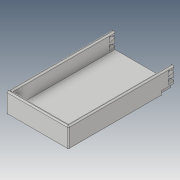
# Autodesk Inventor part: Case_metà1
Saved by Autodesk Inventor 2019 (Build 230136000, 136)
## iProperties
Created: 2019-05-06
Part Number: Case_metà1
Material: Generic
Document SubType Name: Modeling
Designer: giacomo
Density: 1 g/cm^3
Appearance: Default
Author: giacomo
Autodesk Inventor part; units mm, degrees
ref_plane "YZ Plane" through (0, 0, 0) normal (1, 0, 0) x (0, 1, 0)
ref_plane "XZ Plane" through (0, 0, 0) normal (0, 1, 0) x (-1, 0, 0)
ref_plane "XY Plane" through (0, 0, 0) normal (0, 0, 1) x (1, 0, 0)
sketch "Sketch1" plane through (0, 0, 0) normal (0, 1, 0) x (-1, 0, 0)
  line L0 (-50, 75) -> (50, 75)
  line L1 (50, 75) -> (50, -75)
  line L2 (50, -75) -> (-50, -75)
  line L3 (-50, -75) -> (-50, 75)
  line L4 (-50, 75) -> (50, -75) construction
  line L5 (50, 75) -> (-50, -75) construction
  point P0 (0, 0)
  dimension "d0" = 100
  dimension "d1" = 150
  constraints: 12 end point, 2 midpoint, 2 parallel, 1 horizontal, 1 perpendicular
  measures "d0" distance of L1.end L2.end
  measures "d1" distance of L0.end L1.end
extrude "Extrusion1" add sketch "Sketch1" along normal blind 8
sketch "Sketch3" plane through (0, 8, 0) normal (0, 1, 0) x (1, 0, 0)
  line L0 (-50, -75) -> (50, -75) projected
  line L1 (50, -75) -> (50, 75) projected
  line L2 (50, 75) -> (-50, 75) projected
  line L3 (-50, 75) -> (-50, -75) projected
  line L4 (45, 75) -> (45, -70)
  line L5 (-50, -75) -> (50, -75) projected
  line L6 (50, -75) -> (50, 75) projected
  line L7 (0, 0) -> (0, -83) construction
  line L8 (-45, 75) -> (-45, -70)
  line L9 (45, -70) -> (-45, -70)
  dimension "d4" = 5
  dimension "d5" = 5
  constraints: 8 end point, 3 parallel, 2 point on line, 1 perpendicular, 1 vertical, 1 other
  measures "d4" distance between parallel lines of L1 L4
  measures "d5" distance between parallel lines of L9 L0
extrude "Extrusion2" add sketch "Sketch3" along normal blind 25 contours L3 L2 L8 L9 L4 L1 L0
sketch "Sketch4" plane through (50, 0, -75) normal (0, 0, -1) x (-1, 0, 0)
  line L0 (100, 0) -> (0, 0) projected
  line L1 (100, 0) -> (100, 33) projected
  line L2 (95, 33) -> (100, 33) projected
  line L3 (95, 8) -> (95, 33) projected
  line L4 (5, 8) -> (95, 8) projected
  line L5 (5, 8) -> (5, 33) projected
  line L6 (0, 33) -> (5, 33) projected
  line L7 (0, 0) -> (0, 33) projected
  line L8 (95, 8) -> (5, 8) projected
  line L9 (5, 8) -> (5, 0)
  line L10 (95, 8) -> (95, 0)
  line L11 (0, 0) -> (100, 0) projected
  line L12 (0, 0) -> (0, 33) projected
  line L13 (5, 3) -> (95, 3)
  line L14 (5, 8) -> (95, 8) projected
  line L15 (5, 6) -> (95, 6)
  line L16 (5, 8) -> (0, 8)
  line L17 (100, 0) -> (0, 0) projected
  point P0 (50, 0)
  dimension "d8" = 3
  dimension "d9" = 3
  constraints: 10 end point, 8 point on line, 6 parallel, 2 perpendicular, 1 vertical
  measures "d8" distance between parallel lines of L0 L13
  measures "d9" distance between parallel lines of L13 L15
extrude "Extrusion3" add sketch "Sketch4" along normal blind 20 contours L0 L10 L3 L2 L1 | L0 L9 L13 L10 | L15 L9 L4 L10 | L7 L6 L5 L16
sketch "Sketch6" plane through (50, 0, 75) normal (1, 0, 0) x (0, 0, -1)
  line L0 (150, 0) -> (150, 8)
  line L1 (170, 33) -> (170, 8)
  line L2 (0, 0) -> (0, 33) projected
  line L3 (150, 8) -> (170, 8)
  line L4 (170, 33) -> (170, 8) projected
  line L5 (170, 13) -> (161, 10.5)
  line L6 (161, 10.5) -> (161, 19)
  line L7 (161, 19) -> (170, 16.5)
  line L8 (170, 24.5) -> (161, 22)
  line L9 (161, 22) -> (161, 30)
  line L10 (161, 30) -> (170, 28)
  line L11 (170, 28) -> (170, 24.5)
  line L12 (170, 16.5) -> (170, 13)
  point P0 (75, 0)
  dimension "d14" = 3.5
  dimension "d15" = 9
  dimension "d16" = 2.5
  dimension "d17" = 2.5
  dimension "d18" = 3.5
  dimension "d19" = 2.5
  dimension "d20" = 2
  dimension "d21" = 8
  dimension "d22" = 9
  constraints: 22 end point, 2 point on line, 2 vertical, 1 collinear, 1 parallel
  measures "d14" distance of L5.start L7.end
  measures "d15" distance between parallel lines of L1 L6
  measures "d16" vertical distance of L5.end L5.start
  measures "d17" vertical distance of L6.end L7.end
  measures "d18" distance of L8.start L10.end
  measures "d19" vertical distance of L8.end L8.start
  measures "d20" vertical distance of L10.start L10.end
  measures "d21" distance of L7.end L8.start
  measures "d22" distance between parallel lines of L4 L9
extrude "Extrusion4" cut sketch "Sketch6" against normal through all
fillet "Fillet1" radius 2 11 edges at (50, 0, 0) (50, 33, -10) (50, 16.5, 75) (0, 33, 75) (0, 0, 75) (-50, 33, -10) (-50, 16.5, 75) (-50, 0, -10) (45, 33, -12.5) (-45, 33, -12.5) (0, 33, 70)
body "Solid1"
